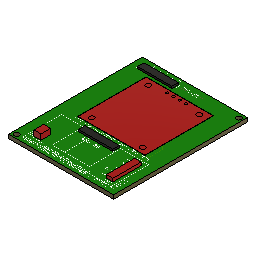
Kube-Module-Enclosure-Submodule-OLED (Autodesk Fusion 360 archive; units mm, degrees)
design "Kube-Module-OLED_AmbiMate"
part number: DISPLAY-OLED-128X64-I2C
Autodesk Fusion 360 part; units mm, degrees
sketch "sketch 296" plane through (0, 0, 0) normal (0, 0, 1) x (1, 0, 0)
  line L0 (16.51, 10.16) -> (59.36, 10.16)
  line L1 (59.36, 10.16) -> (59.36, 64.76)
  line L2 (59.36, 64.76) -> (16.51, 64.76)
  line L3 (16.51, 64.76) -> (16.51, 10.16)
  circle A0 centre (57.785, 62.865) radius 1
  circle A1 centre (18.232, 11.72) radius 1
extrude "Board" add sketch "sketch 296" along normal blind 1.57 makes body 1 in component "Board"
sketch "sketch 8875" plane through (0, 0, 0) normal (0, 0, 1) x (1, 0, 0)
  line L0 (-13.716, -13.97) -> (13.716, -13.97)
  line L1 (13.716, -13.97) -> (13.716, 13.97)
  line L2 (13.716, 13.97) -> (-13.716, 13.97)
  line L3 (-13.716, 13.97) -> (-13.716, -13.97)
extrude "DISPLAY-OLED-128X64-I2C" add sketch "sketch 8875" along normal blind 0.1 separate body makes body 2 in component "DISPLAY-OLED-128X64-I2C"
sketch "sketch 9603" plane through (0, 0, 0) normal (0, 0, 1) x (1, 0, 0)
  line L0 (-2.1082, 0.8001) -> (2.1082, 0.8001)
  line L1 (2.1082, 0.8001) -> (2.1082, -0.8001)
  line L2 (2.1082, -0.8001) -> (-2.1082, -0.8001)
  line L3 (-2.1082, -0.8001) -> (-2.1082, 0.8001)
extrude "SJ_2" add sketch "sketch 9603" along normal blind 2.176 separate body makes body 3 in component "SJ_2"
sketch "sketch 9743" plane through (0, 0, 0) normal (0, 0, 1) x (1, 0, 0)
  line L0 (-7.0104, 1.3208) -> (7.0104, 1.3208)
  line L1 (7.0104, 1.3208) -> (7.0104, -1.3208)
  line L2 (7.0104, -1.3208) -> (-7.0104, -1.3208)
  line L3 (-7.0104, -1.3208) -> (-7.0104, 1.3208)
extrude "FE06" add sketch "sketch 9743" along normal blind 0.778 separate body makes body 4 in component "FE06"
sketch "sketch 9875" plane through (0, 0, 0) normal (0, 0, 1) x (1, 0, 0)
  line L0 (-5.7404, 1.3208) -> (5.7404, 1.3208)
  line L1 (5.7404, 1.3208) -> (5.7404, -1.3208)
  line L2 (5.7404, -1.3208) -> (-5.7404, -1.3208)
  line L3 (-5.7404, -1.3208) -> (-5.7404, 1.3208)
extrude "FE05-1" add sketch "sketch 9875" along normal blind 1.291 separate body makes body 5 in component "FE05-1"
sketch "sketch 10007" plane through (0, 0, 0) normal (0, 0, 1) x (1, 0, 0)
  line L0 (-1.4224, 1.9812) -> (1.4224, 1.9812)
  line L1 (1.4224, 1.9812) -> (1.4224, -1.9812)
  line L2 (1.4224, -1.9812) -> (-1.4224, -1.9812)
  line L3 (-1.4224, -1.9812) -> (-1.4224, 1.9812)
extrude "JP1" add sketch "sketch 10007" along normal blind 2.265 separate body makes body 6 in component "JP1"
sketch "sketch 9295" plane through (0, 0, 0) normal (0, 0, 1) x (1, 0, 0)
  circle A0 centre (20.32, 60.96) radius 0.4065
  circle A1 centre (22.86, 60.96) radius 0.4065
  circle A2 centre (25.4, 60.96) radius 0.4065
  circle A3 centre (27.94, 60.96) radius 0.4065
  circle A4 centre (30.48, 60.96) radius 0.4065
  circle A5 centre (33.02, 60.96) radius 0.4065
  circle A6 centre (30.48, 26.67) radius 0.4065
  circle A7 centre (33.02, 26.67) radius 0.4065
  circle A8 centre (35.56, 26.67) radius 0.4065
  circle A9 centre (38.1, 26.67) radius 0.4065
  circle A10 centre (40.64, 26.67) radius 0.4065
  circle A11 centre (43.18, 26.67) radius 0.4065
  circle A12 centre (34.29, 57.15) radius 0.5
  circle A13 centre (36.83, 57.15) radius 0.5
  circle A14 centre (39.37, 57.15) radius 0.5
  circle A15 centre (41.91, 57.15) radius 0.5
  circle A16 centre (27.686, 56.007) radius 1
  circle A17 centre (48.514, 56.007) radius 1
  circle A18 centre (48.514, 32.893) radius 1
  circle A19 centre (27.686, 32.893) radius 1
  circle A20 centre (53.34, 25.4) radius 0.4065
  circle A21 centre (53.34, 22.86) radius 0.4065
  circle A22 centre (53.34, 20.32) radius 0.4065
  circle A23 centre (53.34, 17.78) radius 0.4065
  circle A24 centre (53.34, 15.24) radius 0.4065
  circle A25 centre (23.838, 15.283) radius 0.457
  circle A26 centre (23.838, 17.823) radius 0.457
extrude "Extrude12" cut sketch "sketch 9295" along normal blind 1.57 bodies 1 in component "Board"
component "PCB Component" placed x (1, 0, 0) y (0, 1, 0) z (0, 0, 1) at (0, 0, 0)
component "Board" placed x (1, 0, 0) y (0, 1, 0) z (0, 0, 1) at (0, 0, 0) in component "PCB Component"
component "DISPLAY-OLED-128X64-I2C" placed x (1, 0, 0) y (0, 1, 0) z (0, 0, 1) at (38.1, 44.45, 1.57) in component "PCB Component"
component "SJ_2" placed x (-1, 0, 0) y (0, 1, 0) z (0, 0, -1) at (26.67, 50.8, 0) in component "PCB Component"
component "SJ_2" placed x (-1, 0, 0) y (0, 1, 0) z (0, 0, -1) at (34.29, 50.8, 0) in component "PCB Component"
component "SJ_2" placed x (-1, 0, 0) y (0, 1, 0) z (0, 0, -1) at (41.91, 50.8, 0) in component "PCB Component"
component "SJ_2" placed x (-1, 0, 0) y (0, 1, 0) z (0, 0, -1) at (49.53, 50.8, 0) in component "PCB Component"
component "SJ_2" placed x (-1, 0, 0) y (0, 1, 0) z (0, 0, -1) at (38.1, 20.32, 0) in component "PCB Component"
component "FE06" placed x (1, 0, 0) y (0, 1, 0) z (0, 0, 1) at (26.67, 60.96, 1.57) in component "PCB Component"
component "FE06" placed x (1, 0, 0) y (0, 1, 0) z (0, 0, 1) at (36.83, 26.67, 1.57) in component "PCB Component"
component "FE05-1" placed x (0, -1, 0) y (1, 0, 0) z (0, 0, 1) at (53.34, 20.32, 1.57) in component "PCB Component"
component "JP1" placed x (1, 0, 0) y (0, 1, 0) z (0, 0, 1) at (23.838, 16.553, 1.57) in component "PCB Component"
named bodies: "Board", "DISPLAY-OLED-128X64-I2C", "SJ_2", "FE06", "FE05-1", "JP1"
